Autodesk Fusion 360 part; units mm, degrees
(part 2 of 2)
  line L749 (33.9, 0.2048) -> (33.9, 2.8393) construction
  line L750 (33.9, 2.8393) -> (36.5607, 5.5) construction
  line L751 (-33.9, 2.8393) -> (-33.9, 0.2048) construction
  line L752 (14.4619, 9.8746) -> (14.4312, 9.8494) construction
  line L753 (14.6743, 9.9793) -> (14.6363, 9.9678) construction
  line L754 (14.9, 10) -> (14.7917, 9.9987) construction
  line L755 (38.2, 5.5) -> (38.2, 3.2628) construction
  arc A45 (-38.5414, 3.1214) -> (-38.2, 3.2628) centre (-38.4, 3.2628) ccw construction
  line L756 (14.5991, 9.9538) -> (14.563, 9.9374) construction
  line L757 (36.5607, 5.5) -> (38.2, 5.5) construction
  line L758 (14.713, 9.9883) -> (14.6743, 9.9793) construction
  line L759 (-36.5607, 5.5) -> (-33.9, 2.8393) construction
  line L760 (-38.2, 3.2628) -> (-38.2, 5.5) construction
  line L761 (14.4022, 9.8222) -> (13.1214, 8.5414) construction
  line L762 (4.5, 6.5607) -> (4.5, 8.2) construction
  line L763 (5.3637, -9.9678) -> (5.4009, -9.9538) construction
  line L764 (-40, 9.5) -> (-40, 8.5) construction
  line L765 (5.3637, 9.9678) -> (5.3257, 9.9793) construction
  line L766 (-34.4942, 9.8977) -> (-34.5279, 9.9187) construction
  line L767 (5.5058, 9.8977) -> (5.4721, 9.9187) construction
  line L768 (6.8786, 8.5414) -> (5.5978, 9.8222) construction
  line L769 (33.2628, 8.2) -> (35.5, 8.2) construction
  line L770 (2.7, -6.2393) -> (2.7, -8.2) construction
  line L771 (34.5279, 9.9187) -> (34.4942, 9.8977) construction
  line L772 (5.4009, -9.9538) -> (5.437, -9.9374) construction
  line L773 (6.1, -0.207) -> (6.1, -2.8393) construction
  line L774 (-34.5279, 9.9187) -> (-34.563, 9.9374) construction
  line L775 (34.4312, 9.8494) -> (34.4022, 9.8222) construction
  line L776 (10.1999, 3.9) -> (10, 3.7001) construction
  line L777 (34.4942, 9.8977) -> (34.4619, 9.8746) construction
  line L778 (6.7372, -8.2) -> (4.5, -8.2) construction
  line L779 (34.4022, 9.8222) -> (33.1214, 8.5414) construction
  line L780 (-34.4022, 9.8222) -> (-34.4312, 9.8494) construction
  line L781 (-33.1214, 8.5414) -> (-34.4022, 9.8222) construction
  line L782 (-34.4619, 9.8746) -> (-34.4942, 9.8977) construction
  line L783 (34.4619, 9.8746) -> (34.4312, 9.8494) construction
  line L784 (34.563, 9.9374) -> (34.5279, 9.9187) construction
  line L785 (-34.4312, 9.8494) -> (-34.4619, 9.8746) construction
  line L786 (35.5, 8.2) -> (35.5, 6.5607) construction
  arc A46 (6.8786, -8.5414) -> (6.7372, -8.2) centre (6.7372, -8.4) ccw construction
  arc A47 (-39.5, 10) -> (-40, 9.5) centre (-39.5, 9.5) ccw construction
  line L787 (4.5, -8.2) -> (4.5, -6.5607) construction
  line L788 (-34.6363, -9.9678) -> (-34.5991, -9.9538) construction
  line L789 (-34.4022, -9.8222) -> (-33.1214, -8.5414) construction
  line L790 (-34.5991, -9.9538) -> (-34.563, -9.9374) construction
  line L791 (-34.713, -9.9883) -> (-34.6743, -9.9793) construction
  line L792 (-33.2628, -8.2) -> (-35.5, -8.2) construction
  line L793 (25.4009, 9.9538) -> (25.3637, 9.9678) construction
  line L794 (-34.7917, -9.9987) -> (-34.7522, -9.9948) construction
  line L795 (25.5688, 9.8494) -> (25.5381, 9.8746) construction
  line L796 (-25.5978, 9.8222) -> (-26.8786, 8.5414) construction
  line L797 (-39.5, -10) -> (-38.5, -10) construction
  line L798 (-34.4312, -9.8494) -> (-34.4022, -9.8222) construction
  line L799 (-38.5, -10) -> (-34.8314, -10) construction
  line L800 (-26.7372, 8.2) -> (-24.5, 8.2) construction
  arc A48 (-26.8786, 8.5414) -> (-26.7372, 8.2) centre (-26.7372, 8.4) ccw construction
  line L801 (-34.4619, -9.8746) -> (-34.4312, -9.8494) construction
  line L802 (25.5381, 9.8746) -> (25.5058, 9.8977) construction
  line L803 (25.5058, 9.8977) -> (25.4721, 9.9187) construction
  line L804 (-34.7522, -9.9948) -> (-34.713, -9.9883) construction
  line L805 (-25.5688, 9.8494) -> (-25.5978, 9.8222) construction
  line L806 (-34.6743, -9.9793) -> (-34.6363, -9.9678) construction
  line L807 (25.4721, 9.9187) -> (25.437, 9.9374) construction
  line L808 (-34.5279, -9.9187) -> (-34.4942, -9.8977) construction
  line L809 (25.437, 9.9374) -> (25.4009, 9.9538) construction
  line L810 (-34.8314, -10) -> (-34.7917, -9.9987) construction
  arc A49 (-40, -9.5) -> (-39.5, -10) centre (-39.5, -9.5) ccw construction
  line L811 (25.3257, 9.9793) -> (25.287, 9.9883) construction
  arc A50 (-33.1214, -8.5414) -> (-33.2628, -8.2) centre (-33.2628, -8.4) ccw construction
  line L812 (25.3637, 9.9678) -> (25.3257, 9.9793) construction
  line L813 (-34.563, -9.9374) -> (-34.5279, -9.9187) construction
  line L814 (-24.5, 8.2) -> (-24.5, 6.5607) construction
  line L815 (25.287, 9.9883) -> (25.2478, 9.9948) construction
  line L816 (-33.9, -0.207) -> (-33.9, -2.8393) construction
  circle A51 centre (-30, 0) radius 2.1 construction
  line L817 (-29.8001, 3.9) -> (-30, 3.7001) construction
  line L818 (-26.1, -2.8393) -> (-26.1, -0.207) construction
  line L819 (-24.5, 6.5607) -> (-27.1607, 3.9) construction
  line L820 (24.5, 6.5607) -> (24.5, 8.2) construction
  line L821 (-40, -4.8314) -> (-40, -8.5) construction
  arc A52 (26.7372, 8.2) -> (26.8786, 8.5414) centre (26.7372, 8.4) ccw construction
  line L822 (-14.9, 10) -> (-25.1, 10) construction
  line L823 (30.1999, 3.9) -> (30, 3.7001) construction
  line L824 (5.5978, 9.8222) -> (5.5688, 9.8494) construction
  line L825 (30, 3.7001) -> (29.8001, 3.9) construction
  line L826 (-30, 3.7001) -> (-30.1999, 3.9) construction
  line L827 (22.7, 8.2) -> (22.7, 6.2393) construction
  line L828 (-26.1, 0.207) -> (-26.1, 2.8393) construction
  line L829 (25.2083, 9.9987) -> (25.1, 10) construction
  line L830 (5.5688, 9.8494) -> (5.5381, 9.8746) construction
  line L831 (27.1607, 3.9) -> (24.5, 6.5607) construction
  line L832 (-26.1, 2.8393) -> (-22.7, 6.2393) construction
  line L833 (-22.7, 6.2393) -> (-22.7, 8.2) construction
  line L834 (-40, -8.5) -> (-40, -9.5) construction
  line L835 (-22.7, 8.2) -> (-17.3, 8.2) construction
  line L836 (-35.5, -8.2) -> (-35.5, -6.5607) construction
  line L837 (-32.8393, -3.9) -> (-30.1999, -3.9) construction
  line L838 (-30.1999, 3.9) -> (-32.8393, 3.9) construction
  line L839 (32.8393, 3.9) -> (30.1999, 3.9) construction
  line L840 (-25.1, -10) -> (-14.9, -10) construction
  line L841 (25.2478, 9.9948) -> (25.2083, 9.9987) construction
  line L842 (-27.1607, 3.9) -> (-29.8001, 3.9) construction
  line L843 (-17.3, -8.2) -> (-22.7, -8.2) construction
  line L844 (29.8001, 3.9) -> (27.1607, 3.9) construction
  line L845 (26.1, 2.8393) -> (26.1, 0.207) construction
  line L846 (9.8001, 3.9) -> (7.1607, 3.9) construction
  line L847 (22.7, 6.2393) -> (26.1, 2.8393) construction
  line L848 (-34.6743, 9.9793) -> (-34.713, 9.9883) construction
  line L849 (5.2478, 9.9948) -> (5.2083, 9.9987) construction
  line L850 (-34.563, 9.9374) -> (-34.5991, 9.9538) construction
  line L851 (7.1607, 3.9) -> (4.5, 6.5607) construction
  line L852 (-34.7917, 9.9987) -> (-34.9, 10) construction
  line L853 (-34.6363, 9.9678) -> (-34.6743, 9.9793) construction
  line L854 (-34.5991, 9.9538) -> (-34.6363, 9.9678) construction
  line L855 (5.4009, 9.9538) -> (5.3637, 9.9678) construction
  line L856 (5.3257, 9.9793) -> (5.287, 9.9883) construction
  line L857 (5.5381, 9.8746) -> (5.5058, 9.8977) construction
  line L858 (5.287, 9.9883) -> (5.2478, 9.9948) construction
  line L859 (-34.713, 9.9883) -> (-34.7522, 9.9948) construction
  line L860 (5.4721, 9.9187) -> (5.437, 9.9374) construction
  arc A53 (-33.2628, 8.2) -> (-33.1214, 8.5414) centre (-33.2628, 8.4) ccw construction
  line L861 (5.437, 9.9374) -> (5.4009, 9.9538) construction
  line L862 (2.7, 8.2) -> (2.7, 6.2393) construction
  line L863 (-34.7522, 9.9948) -> (-34.7917, 9.9987) construction
  arc A54 (6.7372, 8.2) -> (6.8786, 8.5414) centre (6.7372, 8.4) ccw construction
  line L864 (5.2083, 9.9987) -> (5.1, 10) construction
  line L865 (4.5, 8.2) -> (6.7372, 8.2) construction
  arc A55 (33.1214, 8.5414) -> (33.2628, 8.2) centre (33.2628, 8.4) ccw construction
  line L866 (10, 3.7001) -> (9.8001, 3.9) construction
  line L867 (2.7, 6.2393) -> (6.1, 2.8393) construction
  line L868 (-36.5607, 5.5) -> (-33.9, 2.8393)
  line L869 (-36.5607, 5.5) -> (-38.2, 5.5)
  line L870 (-38.2, 5.5) -> (-38.2, 3.2628)
  line L871 (-35.5, 8.2) -> (-35.5, 6.5607)
  line L872 (-35.5, 6.5607) -> (-32.8393, 3.9)
  line L873 (-35.5, 8.2) -> (-33.2628, 8.2)
  line L874 (-40, 9.5) -> (-39.9987, 4.7917)
  line L875 (-39.5, 10) -> (-34.9, 10)
  line L876 (-34.4022, 9.8222) -> (-33.1214, 8.5414)
  line L877 (-38.5414, 3.1214) -> (-39.8494, 4.4312)
  line L878 (-32.8393, 3.9) -> (-27.1607, 3.9)
  line L879 (-27.1607, 3.9) -> (-24.5, 6.5607)
  line L880 (-24.5, 6.5607) -> (-24.5, 8.2)
  line L881 (-24.5, 8.2) -> (-26.7372, 8.2)
  line L882 (-26.8786, 8.5414) -> (-25.5978, 9.8222)
  line L883 (-22.7, 8.2) -> (-22.7, 6.2393)
  line L884 (-22.7, 6.2393) -> (-26.1, 2.8393)
  line L885 (-33.9, 2.8393) -> (-33.9, -2.8393)
  line L886 (-33.9, -2.8393) -> (-36.5607, -5.5)
  line L887 (-36.5607, -5.5) -> (-38.2, -5.5)
  line L888 (-38.2, -5.5) -> (-38.2, -3.2628)
  line L889 (-38.5414, -3.1214) -> (-39.8494, -4.4312)
  line L890 (-40, -9.5) -> (-40, -4.8314)
  line L891 (-39.5, -10) -> (-34.7917, -9.9987)
  line L892 (-35.5, -8.2) -> (-33.2628, -8.2)
  line L893 (-33.1214, -8.5414) -> (-34.4022, -9.8222)
  line L894 (-35.5, -8.2) -> (-35.5, -6.5607)
  line L895 (-35.5, -6.5607) -> (-32.8393, -3.9)
  line L896 (-32.8393, -3.9) -> (-27.1607, -3.9)
  line L897 (-27.1607, -3.9) -> (-24.5, -6.5607)
  line L898 (-24.5, -6.5607) -> (-24.5, -8.2)
  line L899 (-24.5, -8.2) -> (-26.7372, -8.2)
  line L900 (-26.8786, -8.5414) -> (-25.5688, -9.8494)
  line L901 (-26.1, -2.8393) -> (-22.7, -6.2393)
  line L902 (-22.7, -6.2393) -> (-22.7, -8.2)
  line L903 (-26.1, 2.8393) -> (-26.1, -2.8393)
  line L904 (-15.5, -8.2) -> (-13.2628, -8.2)
  line L905 (-13.1214, -8.5414) -> (-14.4022, -9.8222)
  line L906 (-15.5, -8.2) -> (-15.5, -6.5607)
  line L907 (-15.5, -6.5607) -> (-12.8393, -3.9)
  line L908 (-12.8393, -3.9) -> (-7.1607, -3.9)
  line L909 (-7.1607, -3.9) -> (-4.5, -6.5607)
  line L910 (-4.5, -6.5607) -> (-4.5, -8.2)
  line L911 (-4.5, -8.2) -> (-6.7372, -8.2)
  line L912 (-6.8786, -8.5414) -> (-5.5688, -9.8494)
  line L913 (-13.9, -2.8393) -> (-17.3, -6.2393)
  line L914 (-17.3, -6.2393) -> (-17.3, -8.2)
  line L915 (-17.3, -8.2) -> (-22.7, -8.2)
  line L916 (-13.9, -2.8393) -> (-13.9, 2.8393)
  line L917 (-13.9, 2.8393) -> (-17.3, 6.2393)
  line L918 (-22.7, 8.2) -> (-17.3, 8.2)
  line L919 (-17.3, 8.2) -> (-17.3, 6.2393)
  line L920 (-25.1, 10) -> (-14.9, 10)
  line L921 (-13.1214, 8.5414) -> (-14.4022, 9.8222)
  line L922 (-13.2628, 8.2) -> (-15.5, 8.2)
  line L923 (-15.5, 8.2) -> (-15.5, 6.5607)
  line L924 (-15.5, 6.5607) -> (-12.8393, 3.9)
  line L925 (-12.8393, 3.9) -> (-7.1607, 3.9)
  line L926 (-7.1607, 3.9) -> (-4.5, 6.5607)
  line L927 (-4.5, 6.5607) -> (-4.5, 8.2)
  line L928 (-4.5, 8.2) -> (-6.7372, 8.2)
  line L929 (-6.8786, 8.5414) -> (-5.5978, 9.8222)
  line L930 (-2.7, 8.2) -> (-2.7, 6.2393)
  line L931 (-2.7, 6.2393) -> (-6.1, 2.8393)
  line L932 (-6.1, 2.8393) -> (-6.1, -2.8393)
  line L933 (-6.1, -2.8393) -> (-2.7, -6.2393)
  line L934 (-2.7, -6.2393) -> (-2.7, -8.2)
  line L935 (-2.7, -8.2) -> (2.7, -8.2)
  line L936 (2.7, -8.2) -> (2.7, -6.2393)
  line L937 (-5.2083, 9.9987) -> (5.1, 10)
  line L938 (-2.7, 8.2) -> (2.7, 8.2)
  line L939 (2.7, 8.2) -> (2.7, 6.2393)
  line L940 (2.7, 6.2393) -> (6.1, 2.8393)
  line L941 (6.1, 2.8393) -> (6.1, -2.8393)
  line L942 (6.1, -2.8393) -> (2.7, -6.2393)
  line L943 (-5.1, -10) -> (5.1, -10)
  line L944 (5.5688, -9.8494) -> (6.8786, -8.5414)
  line L945 (6.7372, -8.2) -> (4.5, -8.2)
  line L946 (4.5, -8.2) -> (4.5, -6.5607)
  line L947 (4.5, -6.5607) -> (7.1607, -3.9)
  line L948 (7.1607, -3.9) -> (12.8393, -3.9)
  line L949 (12.8393, -3.9) -> (15.5, -6.5607)
  line L950 (15.5, -6.5607) -> (15.5, -8.2)
  line L951 (15.5, -8.2) -> (13.2628, -8.2)
  line L952 (13.1214, -8.5414) -> (14.4312, -9.8494)
  line L953 (14.9, -10) -> (25.1, -10)
  line L954 (25.5688, -9.8494) -> (26.8786, -8.5414)
  line L955 (26.7372, -8.2) -> (24.5, -8.2)
  line L956 (24.5, -8.2) -> (24.5, -6.5607)
  line L957 (24.5, -6.5607) -> (27.1607, -3.9)
  line L958 (26.1, -2.8393) -> (22.7, -6.2393)
  line L959 (22.7, -8.2) -> (17.3, -8.2)
  line L960 (22.7, -6.2393) -> (22.7, -8.2)
  line L961 (17.3, -8.2) -> (17.3, -6.2393)
  line L962 (17.3, -6.2393) -> (13.9, -2.8393)
  line L963 (13.9, -2.8393) -> (13.9, 2.8393)
  line L964 (13.9, 2.8393) -> (17.3, 6.2393)
  line L965 (17.3, 6.2393) -> (17.3, 8.2)
  line L966 (17.3, 8.2) -> (22.7, 8.2)
  line L967 (22.7, 8.2) -> (22.7, 6.2393)
  line L968 (22.7, 6.2393) -> (26.1, 2.8393)
  line L969 (26.1, 2.8393) -> (26.1, -2.8393)
  line L970 (6.8786, 8.5414) -> (5.5978, 9.8222)
  line L971 (6.7372, 8.2) -> (4.5, 8.2)
  line L972 (4.5, 8.2) -> (4.5, 6.5607)
  line L973 (4.5, 6.5607) -> (7.1607, 3.9)
  line L974 (7.1607, 3.9) -> (12.8393, 3.9)
  line L975 (12.8393, 3.9) -> (15.5, 6.5607)
  line L976 (15.5, 6.5607) -> (15.5, 8.2)
  line L977 (15.5, 8.2) -> (13.2628, 8.2)
  line L978 (13.1214, 8.5414) -> (14.4022, 9.8222)
  line L979 (14.9, 10) -> (25.1, 10)
  line L980 (26.8786, 8.5414) -> (25.5978, 9.8222)
  line L981 (26.7372, 8.2) -> (24.5, 8.2)
  line L982 (24.5, 8.2) -> (24.5, 6.5607)
  line L983 (24.5, 6.5607) -> (27.1607, 3.9)
  line L984 (27.1607, 3.9) -> (32.8393, 3.9)
  line L985 (32.8393, 3.9) -> (35.5, 6.5607)
  line L986 (35.5, 6.5607) -> (35.5, 8.2)
  line L987 (35.5, 8.2) -> (33.2628, 8.2)
  line L988 (33.1214, 8.5414) -> (34.4022, 9.8222)
  line L989 (34.7917, 9.9987) -> (39.5, 10)
  line L990 (40, 9.5) -> (40, 4.8314)
  line L991 (39.8494, 4.4312) -> (38.5414, 3.1214)
  line L992 (38.2, 3.2628) -> (38.2, 5.5)
  line L993 (38.2, 5.5) -> (36.5607, 5.5)
  line L994 (36.5607, 5.5) -> (33.9, 2.8393)
  line L995 (33.9, 2.8393) -> (33.9, -2.8393)
  line L996 (33.9, -2.8393) -> (36.5607, -5.5)
  line L997 (36.5607, -5.5) -> (38.2, -5.5)
  line L998 (38.2, -5.5) -> (38.2, -3.2628)
  line L999 (38.5414, -3.1214) -> (39.8222, -4.4022)
  line L1000 (39.9987, -4.7917) -> (40, -9.5)
  line L1001 (39.5, -10) -> (34.8314, -10)
  line L1002 (34.4022, -9.8222) -> (33.1214, -8.5414)
  line L1003 (33.2628, -8.2) -> (35.5, -8.2)
  line L1004 (35.5, -8.2) -> (35.5, -6.5607)
  line L1005 (35.5, -6.5607) -> (32.8393, -3.9)
  line L1006 (32.8393, -3.9) -> (27.1607, -3.9)
  arc A56 (38.5414, -3.1214) -> (38.2, -3.2628) centre (38.4, -3.2628) ccw
  arc A57 (40, -4.8314) -> (39.8222, -4.4022) centre (39.3929, -4.8314) ccw
  arc A58 (39.5, -10) -> (40, -9.5) centre (39.5, -9.5) ccw
  arc A59 (34.4022, -9.8222) -> (34.8314, -10) centre (34.8314, -9.3929) ccw
  arc A60 (33.2628, -8.2) -> (33.1214, -8.5414) centre (33.2628, -8.4) ccw
  arc A61 (26.8786, -8.5414) -> (26.7372, -8.2) centre (26.7372, -8.4) ccw
  arc A62 (14.4312, -9.8494) -> (14.9, -10) centre (14.8411, -9.3785) ccw
  arc A63 (13.2628, -8.2) -> (13.1214, -8.5414) centre (13.2628, -8.4) ccw
  arc A64 (6.8786, -8.5414) -> (6.7372, -8.2) centre (6.7372, -8.4) ccw
  arc A65 (-5.5688, -9.8494) -> (-5.1, -10) centre (-5.156, -9.3694) ccw
  arc A66 (-6.7372, -8.2) -> (-6.8786, -8.5414) centre (-6.7372, -8.4) ccw
  arc A67 (-13.1214, -8.5414) -> (-13.2628, -8.2) centre (-13.2628, -8.4) ccw
  arc A68 (-26.7372, -8.2) -> (-26.8786, -8.5414) centre (-26.7372, -8.4) ccw
  arc A69 (-33.1214, -8.5414) -> (-33.2628, -8.2) centre (-33.2628, -8.4) ccw
  arc A70 (-40, -9.5) -> (-39.5, -10) centre (-39.5, -9.5) ccw
  arc A71 (-39.8494, -4.4312) -> (-40, -4.8314) centre (-39.3929, -4.8314) ccw
  arc A72 (-38.2, -3.2628) -> (-38.5414, -3.1214) centre (-38.4, -3.2628) ccw
  arc A73 (-39.5, 10) -> (-40, 9.5) centre (-39.5, 9.5) ccw
  arc A74 (-39.9987, 4.7917) -> (-39.8494, 4.4312) centre (-39.3929, 4.8314) ccw
  arc A75 (-38.5414, 3.1214) -> (-38.2, 3.2628) centre (-38.4, 3.2628) ccw
  arc A76 (-33.2628, 8.2) -> (-33.1214, 8.5414) centre (-33.2628, 8.4) ccw
  arc A77 (-34.4022, 9.8222) -> (-34.9, 10) centre (-34.8425, 9.3751) ccw
  arc A78 (-26.8786, 8.5414) -> (-26.7372, 8.2) centre (-26.7372, 8.4) ccw
  arc A79 (-25.1, 10) -> (-25.5978, 9.8222) centre (-25.1562, 9.3715) ccw
  arc A80 (-14.4022, 9.8222) -> (-14.9, 10) centre (-14.8409, 9.3798) ccw
  arc A81 (-13.2628, 8.2) -> (-13.1214, 8.5414) centre (-13.2628, 8.4) ccw
  arc A82 (-6.8786, 8.5414) -> (-6.7372, 8.2) centre (-6.7372, 8.4) ccw
  arc A83 (-5.2083, 9.9987) -> (-5.5978, 9.8222) centre (-5.1686, 9.3929) ccw
  arc A84 (6.7372, 8.2) -> (6.8786, 8.5414) centre (6.7372, 8.4) ccw
  arc A85 (13.1214, 8.5414) -> (13.2628, 8.2) centre (13.2628, 8.4) ccw
  arc A86 (14.9, 10) -> (14.4022, 9.8222) centre (14.8409, 9.3798) ccw
  arc A87 (25.5978, 9.8222) -> (25.1, 10) centre (25.1575, 9.3751) ccw
  arc A88 (26.7372, 8.2) -> (26.8786, 8.5414) centre (26.7372, 8.4) ccw
  arc A89 (33.1214, 8.5414) -> (33.2628, 8.2) centre (33.2628, 8.4) ccw
  arc A90 (40, 9.5) -> (39.5, 10) centre (39.5, 9.5) ccw
  arc A91 (39.8494, 4.4312) -> (40, 4.8314) centre (39.3929, 4.8314) ccw
  arc A92 (38.2, 3.2628) -> (38.5414, 3.1214) centre (38.4, 3.2628) ccw
  line L1007 (34.4022, 9.8222) -> (34.4312, 9.8494)
  arc A93 (34.7917, 9.9987) -> (34.4312, 9.8494) centre (34.8314, 9.3929) ccw
  arc A94 (25.1, -10) -> (25.5688, -9.8494) centre (25.1572, -9.3734) ccw
  arc A95 (5.1, -10) -> (5.5688, -9.8494) centre (5.1438, -9.3315) ccw
  arc A96 (-14.9, -10) -> (-14.4022, -9.8222) centre (-14.8424, -9.3755) ccw
  line L1008 (-14.9, -10) -> (-25.2083, -9.9987)
  arc A97 (-25.5688, -9.8494) -> (-25.2083, -9.9987) centre (-25.1662, -9.3872) ccw
  arc A98 (-34.7917, -9.9987) -> (-34.4022, -9.8222) centre (-34.8336, -9.3881) ccw
  arc A99 (5.5978, 9.8222) -> (5.1, 10) centre (5.1576, 9.3755) ccw
  circle A100 centre (-30, 0) radius 2.1
  circle A101 centre (-10, 0) radius 2.1
  circle A102 centre (10, 0) radius 2.1
  circle A103 centre (30, 0) radius 2.1
  constraint parallel L472 L868
  constraint parallel L475 L869
  constraint tangent A40 L870
  constraint parallel L695 L871
  constraint parallel L675 L872
  constraint tangent A53 L873
  constraint tangent A37 L876
  constraint parallel L582 L878
  constraint parallel L819 L879
  constraint parallel L814 L880
  constraint tangent A20 L881
  constraint tangent A48 L882
  constraint perpendicular L652 L883
  constraint parallel L832 L884
  constraint parallel L142 L886
  constraint parallel L576 L887
  constraint tangent A6 L888
  constraint tangent A50 L892
  constraint tangent A50 L893
  constraint parallel L836 L894
  constraint parallel L568 L895
  constraint parallel L669 L896
  constraint parallel L532 L897
  constraint parallel L691 L898
  constraint tangent A8 L899
  constraint parallel L525 L901
  constraint perpendicular L843 L902
  constraint tangent A18 L904
  constraint tangent A32 L905
  constraint parallel L542 L906
  constraint parallel L640 L907
  constraint parallel L364 L908
  constraint parallel L395 L909
  constraint parallel L286 L910
  constraint tangent A25 L911
  constraint parallel L530 L913
  constraint perpendicular L843 L914
  constraint perpendicular L502 L915
  constraint perpendicular L915 L916
  constraint parallel L241 L917
  constraint perpendicular L246 L918
  constraint perpendicular L835 L919
  constraint tangent A17 L921
  constraint tangent A17 L922
  constraint parallel L608 L923
  constraint parallel L315 L924
  constraint parallel L371 L925
  constraint parallel L334 L926
  constraint parallel L369 L927
  constraint tangent A22 L928
  constraint tangent A22 L929
  constraint parallel L320 L930
  constraint parallel L335 L931
  constraint parallel L206 L932
  constraint parallel L298 L933
  constraint parallel L302 L934
  constraint parallel L465 L935
  constraint parallel L770 L936
  constraint parallel L432 L938
  constraint parallel L345 L939
  constraint parallel L867 L940
  constraint parallel L773 L941
  constraint parallel L247 L942
  constraint tangent A19 L945
  constraint parallel L787 L946
  constraint parallel L708 L947
  constraint parallel L477 L948
  constraint parallel L470 L949
  constraint parallel L558 L950
  constraint tangent A34 L951
  constraint tangent A3 L955
  constraint parallel L104 L956
  constraint parallel L154 L957
  constraint parallel L115 L958
  constraint perpendicular L680 L959
  constraint perpendicular L959 L960
  constraint perpendicular L959 L961
  constraint parallel L681 L962
  constraint parallel L637 L963
  constraint parallel L194 L964
  constraint perpendicular L654 L965
  constraint perpendicular L827 L966
  constraint perpendicular L966 L967
  constraint parallel L168 L968
  constraint tangent A23 L970
  constraint tangent A23 L971
  constraint parallel L349 L972
  constraint parallel L851 L973
  constraint parallel L629 L974
  constraint parallel L733 L975
  constraint parallel L730 L976
  constraint tangent A44 L977
  constraint tangent A38 L978
  constraint parallel L656 L979
  constraint tangent A5 L980
  constraint tangent A52 L981
  constraint parallel L149 L982
  constraint parallel L56 L983
  constraint parallel L839 L984
  constraint parallel L131 L985
  constraint parallel L786 L986
  constraint tangent A0 L987
  constraint tangent A0 L988
  constraint tangent A12 L992
  constraint parallel L757 L993
  constraint parallel L750 L994
  constraint parallel L415 L996
  constraint parallel L406 L997
  constraint tangent A26 L998
  constraint tangent A11 L999
  constraint tangent A27 L1002
  constraint tangent A30 L1003
  constraint parallel L453 L1004
  constraint parallel L404 L1005
  constraint parallel L157 L1006
  constraint coincident L94.start A57
  constraint coincident L429.start A59
  constraint coincident L504.start A62
  constraint coincident L233.start A65
  constraint coincident L39.start A71
  constraint coincident L484.start A74
  constraint coincident L646.start A77
  constraint coincident L559.end A79
  constraint coincident L204.end A80
  constraint coincident L332.end A83
  constraint coincident L620.end A86
  constraint coincident L44.end A87
  constraint coincident L2.start A91
  constraint parallel L5 L1007
  constraint coincident L12.start A93
  constraint coincident L72.end A94
  constraint tangent L703 A95
  constraint concentric A51 A100
  constraint concentric A14 A101
  constraint concentric A42 A102
  constraint concentric A31 A103
extrude "Extrude1" add sketch "Sketch1" along normal blind 10
sketch "Sketch2" plane through (0, 0, 0) normal (0, 0, -1) x (1, 0, 0)
  line L0 (-2.7, -8.2) -> (-2.7, -6.2393)
  line L1 (-2.7, -6.2393) -> (-6.1, -2.8393)
  line L2 (-6.1, -2.8393) -> (-6.1, 2.8393)
  line L3 (-6.1, 2.8393) -> (-2.7, 6.2393)
  line L4 (-2.7, 6.2393) -> (-2.7, 8.2)
  line L5 (-2.7, 8.2) -> (2.7, 8.2)
  line L6 (2.7, 8.2) -> (2.7, 6.2393)
  line L7 (2.7, 6.2393) -> (6.1, 2.8393)
  line L8 (6.1, 2.8393) -> (6.1, -2.8393)
  line L9 (6.1, -2.8393) -> (2.7, -6.2393)
  line L10 (2.7, -6.2393) -> (2.7, -8.2)
  line L11 (2.7, -8.2) -> (-2.7, -8.2)
  circle A0 centre (-30, 0) radius 2.1
  circle A1 centre (30, 0) radius 2.1
  line L12 (-22.7, -8.2) -> (-22.7, -6.2393)
  line L13 (-22.7, -6.2393) -> (-26.1, -2.8393)
  line L14 (-26.1, -2.8393) -> (-26.1, 2.8393)
  line L15 (-26.1, 2.8393) -> (-22.7, 6.2393)
  line L16 (-22.7, 6.2393) -> (-22.7, 8.2)
  line L17 (-22.7, 8.2) -> (-17.3, 8.2)
  line L18 (-17.3, 8.2) -> (-17.3, 6.2393)
  line L19 (-17.3, 6.2393) -> (-13.9, 2.8393)
  line L20 (-13.9, 2.8393) -> (-13.9, -2.8393)
  line L21 (-13.9, -2.8393) -> (-17.3, -6.2393)
  line L22 (-17.3, -6.2393) -> (-17.3, -8.2)
  line L23 (-17.3, -8.2) -> (-22.7, -8.2)
  circle A2 centre (-10, 0) radius 2.1
  circle A3 centre (10, 0) radius 2.1
  line L24 (26.1, -2.8393) -> (22.7, -6.2393)
  line L25 (22.7, -6.2393) -> (22.7, -8.2)
  line L26 (22.7, -8.2) -> (17.3, -8.2)
  line L27 (17.3, -8.2) -> (17.3, -6.2393)
  line L28 (17.3, -6.2393) -> (13.9, -2.8393)
  line L29 (13.9, -2.8393) -> (13.9, 2.8393)
  line L30 (13.9, 2.8393) -> (17.3, 6.2393)
  line L31 (17.3, 6.2393) -> (17.3, 8.2)
  line L32 (17.3, 8.2) -> (22.7, 8.2)
  line L33 (22.7, 8.2) -> (22.7, 6.2393)
  line L34 (22.7, 6.2393) -> (26.1, 2.8393)
  line L35 (26.1, 2.8393) -> (26.1, -2.8393)
  arc A4 (6.8786, -8.5414) -> (6.7372, -8.2) centre (6.7372, -8.4) ccw
  line L36 (6.7372, -8.2) -> (4.5, -8.2)
  line L37 (4.5, -8.2) -> (4.5, -6.5607)
  line L38 (4.5, -6.5607) -> (7.1607, -3.9)
  line L39 (7.1607, -3.9) -> (12.8393, -3.9)
  line L40 (12.8393, -3.9) -> (15.5, -6.5607)
  line L41 (15.5, -6.5607) -> (15.5, -8.2)
  line L42 (15.5, -8.2) -> (13.2628, -8.2)
  arc A5 (13.2628, -8.2) -> (13.1214, -8.5414) centre (13.2628, -8.4) ccw
  line L43 (13.1214, -8.5414) -> (14.4022, -9.8222)
  arc A6 (14.4022, -9.8222) -> (14.9, -10) centre (14.8409, -9.3798) ccw
  line L44 (14.9, -10) -> (25.1, -10)
  arc A7 (25.1, -10) -> (25.5978, -9.8222) centre (25.1575, -9.3751) ccw
  line L45 (25.5978, -9.8222) -> (26.8786, -8.5414)
  arc A8 (26.8786, -8.5414) -> (26.7372, -8.2) centre (26.7372, -8.4) ccw
  line L46 (26.7372, -8.2) -> (24.5, -8.2)
  line L47 (24.5, -8.2) -> (24.5, -6.5607)
  line L48 (24.5, -6.5607) -> (27.1607, -3.9)
  line L49 (27.1607, -3.9) -> (32.8393, -3.9)
  line L50 (32.8393, -3.9) -> (35.5, -6.5607)
  line L51 (35.5, -6.5607) -> (35.5, -8.2)
  line L52 (35.5, -8.2) -> (33.2628, -8.2)
  arc A9 (33.2628, -8.2) -> (33.1214, -8.5414) centre (33.2628, -8.4) ccw
  line L53 (33.1214, -8.5414) -> (34.4022, -9.8222)
  line L54 (34.4022, -9.8222) -> (34.4312, -9.8494)
  arc A10 (34.4312, -9.8494) -> (34.7917, -9.9987) centre (34.8314, -9.3929) ccw
  line L55 (34.7917, -9.9987) -> (39.5, -10)
  arc A11 (39.5, -10) -> (40, -9.5) centre (39.5, -9.5) ccw
  line L56 (40, -9.5) -> (40, -4.8314)
  arc A12 (40, -4.8314) -> (39.8494, -4.4312) centre (39.3929, -4.8314) ccw
  line L57 (39.8494, -4.4312) -> (38.5414, -3.1214)
  arc A13 (38.5414, -3.1214) -> (38.2, -3.2628) centre (38.4, -3.2628) ccw
  line L58 (38.2, -3.2628) -> (38.2, -5.5)
  line L59 (38.2, -5.5) -> (36.5607, -5.5)
  line L60 (36.5607, -5.5) -> (33.9, -2.8393)
  line L61 (33.9, -2.8393) -> (33.9, 2.8393)
  line L62 (33.9, 2.8393) -> (36.5607, 5.5)
  line L63 (36.5607, 5.5) -> (38.2, 5.5)
  line L64 (38.2, 5.5) -> (38.2, 3.2628)
  arc A14 (38.2, 3.2628) -> (38.5414, 3.1214) centre (38.4, 3.2628) ccw
  line L65 (38.5414, 3.1214) -> (39.8222, 4.4022)
  arc A15 (39.8222, 4.4022) -> (39.9987, 4.7917) centre (39.3929, 4.8314) ccw
  line L66 (39.9987, 4.7917) -> (40, 9.5)
  arc A16 (40, 9.5) -> (39.5, 10) centre (39.5, 9.5) ccw
  line L67 (39.5, 10) -> (34.8314, 10)
  arc A17 (34.8314, 10) -> (34.4022, 9.8222) centre (34.8314, 9.3929) ccw
  line L68 (34.4022, 9.8222) -> (33.1214, 8.5414)
  arc A18 (33.1214, 8.5414) -> (33.2628, 8.2) centre (33.2628, 8.4) ccw
  line L69 (33.2628, 8.2) -> (35.5, 8.2)
  line L70 (35.5, 8.2) -> (35.5, 6.5607)
  line L71 (35.5, 6.5607) -> (32.8393, 3.9)
  line L72 (32.8393, 3.9) -> (27.1607, 3.9)
  line L73 (27.1607, 3.9) -> (24.5, 6.5607)
  line L74 (24.5, 6.5607) -> (24.5, 8.2)
  line L75 (24.5, 8.2) -> (26.7372, 8.2)
  arc A19 (26.7372, 8.2) -> (26.8786, 8.5414) centre (26.7372, 8.4) ccw
  line L76 (26.8786, 8.5414) -> (25.5688, 9.8494)
  arc A20 (25.5688, 9.8494) -> (25.1, 10) centre (25.1572, 9.3734) ccw
  line L77 (25.1, 10) -> (14.9, 10)
  arc A21 (14.9, 10) -> (14.4312, 9.8494) centre (14.8411, 9.3785) ccw
  line L78 (14.4312, 9.8494) -> (13.1214, 8.5414)
  arc A22 (13.1214, 8.5414) -> (13.2628, 8.2) centre (13.2628, 8.4) ccw
  line L79 (13.2628, 8.2) -> (15.5, 8.2)
  line L80 (15.5, 8.2) -> (15.5, 6.5607)
  line L81 (15.5, 6.5607) -> (12.8393, 3.9)
  line L82 (12.8393, 3.9) -> (7.1607, 3.9)
  line L83 (7.1607, 3.9) -> (4.5, 6.5607)
  line L84 (4.5, 6.5607) -> (4.5, 8.2)
  line L85 (4.5, 8.2) -> (6.7372, 8.2)
  arc A23 (6.7372, 8.2) -> (6.8786, 8.5414) centre (6.7372, 8.4) ccw
  line L86 (6.8786, 8.5414) -> (5.5688, 9.8494)
  arc A24 (5.5688, 9.8494) -> (5.1, 10) centre (5.1438, 9.3315) ccw
  line L87 (5.1, 10) -> (-5.1, 10)
  arc A25 (-5.1, 10) -> (-5.5688, 9.8494) centre (-5.156, 9.3694) ccw
  line L88 (-5.5688, 9.8494) -> (-6.8786, 8.5414)
  arc A26 (-6.8786, 8.5414) -> (-6.7372, 8.2) centre (-6.7372, 8.4) ccw
  line L89 (-6.7372, 8.2) -> (-4.5, 8.2)
  line L90 (-4.5, 8.2) -> (-4.5, 6.5607)
  line L91 (-4.5, 6.5607) -> (-7.1607, 3.9)
  line L92 (-7.1607, 3.9) -> (-12.8393, 3.9)
  line L93 (-12.8393, 3.9) -> (-15.5, 6.5607)
  line L94 (-15.5, 6.5607) -> (-15.5, 8.2)
  line L95 (-15.5, 8.2) -> (-13.2628, 8.2)
  arc A27 (-13.2628, 8.2) -> (-13.1214, 8.5414) centre (-13.2628, 8.4) ccw
  line L96 (-13.1214, 8.5414) -> (-14.4022, 9.8222)
  arc A28 (-14.4022, 9.8222) -> (-14.9, 10) centre (-14.8424, 9.3755) ccw
  line L97 (-14.9, 10) -> (-25.2083, 9.9987)
  arc A29 (-25.2083, 9.9987) -> (-25.5688, 9.8494) centre (-25.1662, 9.3872) ccw
  line L98 (-25.5688, 9.8494) -> (-26.8786, 8.5414)
  arc A30 (-26.8786, 8.5414) -> (-26.7372, 8.2) centre (-26.7372, 8.4) ccw
  line L99 (-26.7372, 8.2) -> (-24.5, 8.2)
  line L100 (-24.5, 8.2) -> (-24.5, 6.5607)
  line L101 (-24.5, 6.5607) -> (-27.1607, 3.9)
  line L102 (-27.1607, 3.9) -> (-32.8393, 3.9)
  line L103 (-32.8393, 3.9) -> (-35.5, 6.5607)
  line L104 (-35.5, 6.5607) -> (-35.5, 8.2)
  line L105 (-35.5, 8.2) -> (-33.2628, 8.2)
  arc A31 (-33.2628, 8.2) -> (-33.1214, 8.5414) centre (-33.2628, 8.4) ccw
  line L106 (-33.1214, 8.5414) -> (-34.4022, 9.8222)
  arc A32 (-34.4022, 9.8222) -> (-34.7917, 9.9987) centre (-34.8336, 9.3881) ccw
  line L107 (-34.7917, 9.9987) -> (-39.5, 10)
  arc A33 (-39.5, 10) -> (-40, 9.5) centre (-39.5, 9.5) ccw
  line L108 (-40, 9.5) -> (-40, 4.8314)
  arc A34 (-40, 4.8314) -> (-39.8494, 4.4312) centre (-39.3929, 4.8314) ccw
  line L109 (-39.8494, 4.4312) -> (-38.5414, 3.1214)
  arc A35 (-38.5414, 3.1214) -> (-38.2, 3.2628) centre (-38.4, 3.2628) ccw
  line L110 (-38.2, 3.2628) -> (-38.2, 5.5)
  line L111 (-38.2, 5.5) -> (-36.5607, 5.5)
  line L112 (-36.5607, 5.5) -> (-33.9, 2.8393)
  line L113 (-33.9, 2.8393) -> (-33.9, -2.8393)
  line L114 (-33.9, -2.8393) -> (-36.5607, -5.5)
  line L115 (-36.5607, -5.5) -> (-38.2, -5.5)
  line L116 (-38.2, -5.5) -> (-38.2, -3.2628)
  arc A36 (-38.2, -3.2628) -> (-38.5414, -3.1214) centre (-38.4, -3.2628) ccw
  line L117 (-38.5414, -3.1214) -> (-39.8494, -4.4312)
  arc A37 (-39.8494, -4.4312) -> (-39.9987, -4.7917) centre (-39.3929, -4.8314) ccw
  line L118 (-39.9987, -4.7917) -> (-40, -9.5)
  arc A38 (-40, -9.5) -> (-39.5, -10) centre (-39.5, -9.5) ccw
  line L119 (-39.5, -10) -> (-34.9, -10)
  arc A39 (-34.9, -10) -> (-34.4022, -9.8222) centre (-34.8425, -9.3751) ccw
  line L120 (-34.4022, -9.8222) -> (-33.1214, -8.5414)
  arc A40 (-33.1214, -8.5414) -> (-33.2628, -8.2) centre (-33.2628, -8.4) ccw
  line L121 (-33.2628, -8.2) -> (-35.5, -8.2)
  line L122 (-35.5, -8.2) -> (-35.5, -6.5607)
  line L123 (-35.5, -6.5607) -> (-32.8393, -3.9)
  line L124 (-32.8393, -3.9) -> (-27.1607, -3.9)
  line L125 (-27.1607, -3.9) -> (-24.5, -6.5607)
  line L126 (-24.5, -6.5607) -> (-24.5, -8.2)
  line L127 (-24.5, -8.2) -> (-26.7372, -8.2)
  arc A41 (-26.7372, -8.2) -> (-26.8786, -8.5414) centre (-26.7372, -8.4) ccw
  line L128 (-26.8786, -8.5414) -> (-25.5978, -9.8222)
  arc A42 (-25.5978, -9.8222) -> (-25.1, -10) centre (-25.1562, -9.3715) ccw
  line L129 (-25.1, -10) -> (-14.9, -10)
  arc A43 (-14.9, -10) -> (-14.4022, -9.8222) centre (-14.8409, -9.3798) ccw
  line L130 (-14.4022, -9.8222) -> (-13.1214, -8.5414)
  arc A44 (-13.1214, -8.5414) -> (-13.2628, -8.2) centre (-13.2628, -8.4) ccw
  line L131 (-13.2628, -8.2) -> (-15.5, -8.2)
  line L132 (-15.5, -8.2) -> (-15.5, -6.5607)
  line L133 (-15.5, -6.5607) -> (-12.8393, -3.9)
  line L134 (-12.8393, -3.9) -> (-7.1607, -3.9)
  line L135 (-7.1607, -3.9) -> (-4.5, -6.5607)
  line L136 (-4.5, -6.5607) -> (-4.5, -8.2)
  line L137 (-4.5, -8.2) -> (-6.7372, -8.2)
  arc A45 (-6.7372, -8.2) -> (-6.8786, -8.5414) centre (-6.7372, -8.4) ccw
  line L138 (-6.8786, -8.5414) -> (-5.5978, -9.8222)
  arc A46 (-5.5978, -9.8222) -> (-5.2083, -9.9987) centre (-5.1686, -9.3929) ccw
  line L139 (-5.2083, -9.9987) -> (5.1, -10)
  arc A47 (5.1, -10) -> (5.5978, -9.8222) centre (5.1576, -9.3755) ccw
  line L140 (5.5978, -9.8222) -> (6.8786, -8.5414)
